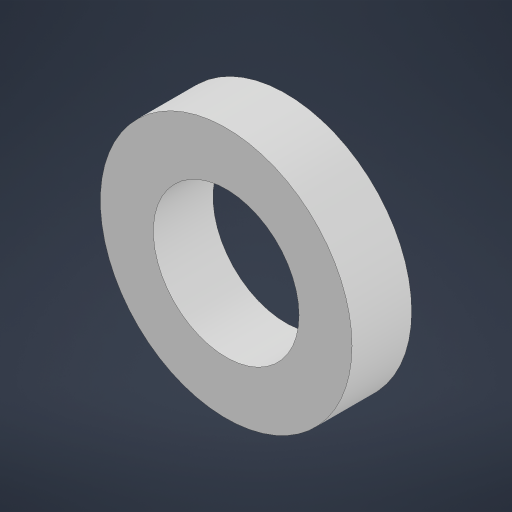
# Autodesk Inventor part: counterbore side
Saved by Autodesk Inventor 2023.2 (Build 272271030, 271C)
## iProperties
Created: 2023-04-05
Part Number: counterbore side
Material: Generic
Document SubType Name: Modeling
Designer: ralph
Density: 1 g/cm^3
Appearance: Default
Author: ralph
Autodesk Inventor part; units mm, degrees
ref_plane "YZ Plane" through (0, 0, 0) normal (1, 0, 0) x (0, 1, 0)
ref_plane "XZ Plane" through (0, 0, 0) normal (0, 1, 0) x (-1, 0, 0)
ref_plane "XY Plane" through (0, 0, 0) normal (0, 0, 1) x (1, 0, 0)
sketch "Sketch1" plane through (0, 0, 0) normal (0, 0, 1) x (1, 0, 0)
  arc A0 (13.9214, 24.4216) -> (10.9603, 25.6482) centre (0, -5) ccw projected
  arc A1 (9.0874, 23.6613) -> (10.9603, 25.6482) centre (2.0185, 32.201) ccw projected
  arc A2 (2.5726, 24.9572) -> (9.0874, 23.6613) centre (6.35, 26.9236) ccw projected
  arc A3 (1.6025, 27.5096) -> (2.5726, 24.9572) centre (12.3713, 30.1417) ccw projected
  arc A4 (1.6025, 27.5096) -> (-1.6025, 27.5096) centre (0, -5) ccw projected
  arc A5 (-2.5726, 24.9572) -> (-1.6025, 27.5096) centre (-12.3713, 30.1417) ccw projected
  arc A6 (-9.0874, 23.6613) -> (-2.5726, 24.9572) centre (-6.35, 26.9236) ccw projected
  arc A7 (-10.9603, 25.6482) -> (-9.0874, 23.6613) centre (-2.0185, 32.201) ccw projected
  arc A8 (-10.9603, 25.6482) -> (-13.9214, 24.4216) centre (0, -5) ccw projected
  arc A9 (-13.8408, 21.6924) -> (-13.9214, 24.4216) centre (-24.8777, 22.7324) ccw projected
  arc A10 (-19.3639, 18.002) -> (-13.8408, 21.6924) centre (-18.0833, 22.0635) ccw projected
  arc A11 (-21.8546, 19.1209) -> (-19.3639, 18.002) centre (-16.1011, 28.5967) ccw projected
  arc A12 (-21.8546, 19.1209) -> (-24.1209, 16.8546) centre (0, -5) ccw projected
  arc A13 (-23.002, 14.3639) -> (-24.1209, 16.8546) centre (-33.5967, 11.1011) ccw projected
  arc A14 (-26.6924, 8.8408) -> (-23.002, 14.3639) centre (-27.0635, 13.0833) ccw projected
  arc A15 (-29.4216, 8.9214) -> (-26.6924, 8.8408) centre (-27.7324, 19.8777) ccw projected
  arc A16 (-29.4216, 8.9214) -> (-30.6482, 5.9603) centre (0, -5) ccw projected
  arc A17 (-28.6613, 4.0874) -> (-30.6482, 5.9603) centre (-37.201, -2.9815) ccw projected
  arc A18 (-29.9572, -2.4274) -> (-28.6613, 4.0874) centre (-31.9236, 1.35) ccw projected
  arc A19 (-32.5096, -3.3975) -> (-29.9572, -2.4274) centre (-35.1417, 7.3713) ccw projected
  arc A20 (-32.5096, -3.3975) -> (-32.5096, -6.6025) centre (0, -5) ccw projected
  arc A21 (-29.9572, -7.5726) -> (-32.5096, -6.6025) centre (-35.1417, -17.3713) ccw projected
  arc A22 (-28.6613, -14.0874) -> (-29.9572, -7.5726) centre (-31.9236, -11.35) ccw projected
  arc A23 (-30.6482, -15.9603) -> (-28.6613, -14.0874) centre (-37.201, -7.0185) ccw projected
  arc A24 (-30.6482, -15.9603) -> (-29.4216, -18.9214) centre (0, -5) ccw projected
  arc A25 (-26.6924, -18.8408) -> (-29.4216, -18.9214) centre (-27.7324, -29.8777) ccw projected
  arc A26 (-23.002, -24.3639) -> (-26.6924, -18.8408) centre (-27.0635, -23.0833) ccw projected
  arc A27 (-24.1209, -26.8546) -> (-23.002, -24.3639) centre (-33.5967, -21.1011) ccw projected
  arc A28 (-24.1209, -26.8546) -> (-21.8546, -29.1209) centre (0, -5) ccw projected
  arc A29 (-19.3639, -28.002) -> (-21.8546, -29.1209) centre (-16.1011, -38.5967) ccw projected
  arc A30 (-13.8408, -31.6924) -> (-19.3639, -28.002) centre (-18.0833, -32.0635) ccw projected
  arc A31 (-13.9214, -34.4216) -> (-13.8408, -31.6924) centre (-24.8777, -32.7324) ccw projected
  arc A32 (-13.9214, -34.4216) -> (-10.9603, -35.6482) centre (0, -5) ccw projected
  arc A33 (-9.0874, -33.6613) -> (-10.9603, -35.6482) centre (-2.0185, -42.201) ccw projected
  arc A34 (-2.5726, -34.9572) -> (-9.0874, -33.6613) centre (-6.35, -36.9236) ccw projected
  arc A35 (-1.6025, -37.5096) -> (-2.5726, -34.9572) centre (-12.3713, -40.1417) ccw projected
  arc A36 (-1.6025, -37.5096) -> (1.6025, -37.5096) centre (0, -5) ccw projected
  arc A37 (2.5726, -34.9572) -> (1.6025, -37.5096) centre (12.3713, -40.1417) ccw projected
  arc A38 (9.0874, -33.6613) -> (2.5726, -34.9572) centre (6.35, -36.9236) ccw projected
  arc A39 (10.9603, -35.6482) -> (9.0874, -33.6613) centre (2.0185, -42.201) ccw projected
  arc A40 (10.9603, -35.6482) -> (13.9214, -34.4216) centre (0, -5) ccw projected
  arc A41 (13.8408, -31.6924) -> (13.9214, -34.4216) centre (24.8777, -32.7324) ccw projected
  arc A42 (19.3639, -28.002) -> (13.8408, -31.6924) centre (18.0833, -32.0635) ccw projected
  arc A43 (21.8546, -29.1209) -> (19.3639, -28.002) centre (16.1011, -38.5967) ccw projected
  arc A44 (21.8546, -29.1209) -> (24.1209, -26.8546) centre (0, -5) ccw projected
  arc A45 (23.002, -24.3639) -> (24.1209, -26.8546) centre (33.5967, -21.1011) ccw projected
  arc A46 (26.6924, -18.8408) -> (23.002, -24.3639) centre (27.0635, -23.0833) ccw projected
  arc A47 (29.4216, -18.9214) -> (26.6924, -18.8408) centre (27.7324, -29.8777) ccw projected
  arc A48 (29.4216, -18.9214) -> (30.6482, -15.9603) centre (0, -5) ccw projected
  arc A49 (28.6613, -14.0874) -> (30.6482, -15.9603) centre (37.201, -7.0185) ccw projected
  arc A50 (29.9572, -7.5726) -> (28.6613, -14.0874) centre (31.9236, -11.35) ccw projected
  arc A51 (32.5096, -6.6025) -> (29.9572, -7.5726) centre (35.1417, -17.3713) ccw projected
  arc A52 (32.5096, -6.6025) -> (32.5096, -3.3975) centre (0, -5) ccw projected
  arc A53 (29.9572, -2.4274) -> (32.5096, -3.3975) centre (35.1417, 7.3713) ccw projected
  arc A54 (28.6613, 4.0874) -> (29.9572, -2.4274) centre (31.9236, 1.35) ccw projected
  arc A55 (30.6482, 5.9603) -> (28.6613, 4.0874) centre (37.201, -2.9815) ccw projected
  arc A56 (30.6482, 5.9603) -> (29.4216, 8.9214) centre (0, -5) ccw projected
  arc A57 (26.6924, 8.8408) -> (29.4216, 8.9214) centre (27.7324, 19.8777) ccw projected
  arc A58 (23.002, 14.3639) -> (26.6924, 8.8408) centre (27.0635, 13.0833) ccw projected
  arc A59 (24.1209, 16.8546) -> (23.002, 14.3639) centre (33.5967, 11.1011) ccw projected
  arc A60 (24.1209, 16.8546) -> (21.8546, 19.1209) centre (0, -5) ccw projected
  arc A61 (19.3639, 18.002) -> (21.8546, 19.1209) centre (16.1011, 28.5967) ccw projected
  arc A62 (13.8408, 21.6924) -> (19.3639, 18.002) centre (18.0833, 22.0635) ccw projected
  arc A63 (13.9214, 24.4216) -> (13.8408, 21.6924) centre (24.8777, 22.7324) ccw projected
  circle A64 centre (0, -5) radius 24.13
  circle A65 centre (0, -5) radius 13.97 projected
  circle A66 centre (0, 14.05) radius 2.3813 projected
  circle A67 centre (19.05, -5) radius 2.3813 projected
  circle A68 centre (-19.05, -5) radius 2.3813 projected
  circle A69 centre (0, -24.05) radius 2.3813 projected
  point P0 (0, 0)
  dimension "d0" = 48.26
  constraints: 1 centre point, 1 coincident
  measures "d0" diameter of A64
extrude "Extrusion1" add sketch "Sketch1" along normal blind 9.525 contours A64 | A65 | A66 | A67 | A68 | A69
sketch "Sketch2" plane through (0, -5, 9.525) normal (0, 0, 1) x (1, 0, 0)
  circle A0 centre (0, 0) radius 24.13 projected
  circle A1 centre (0, 19.05) radius 4.7625
  circle A2 centre (-19.05, 0) radius 1.27 projected
  circle A3 centre (-19.05, 0) radius 4.7625
  circle A4 centre (19.05, 0) radius 4.7625
  circle A5 centre (0, -19.05) radius 4.7625
  point P0 (0, 5)
  dimension "d3" = 9.525
  dimension "d4" = 9.525
  dimension "d5" = 9.525
  dimension "d6" = 9.525
  constraints: 4 centre point, 1 coincident
  measures "d3" diameter of A1
  measures "d4" diameter of A3
  measures "d5" diameter of A4
  measures "d6" diameter of A5
ref_plane "Work Plane1" through (-23.0187, -8.9687, 4.5858) normal (0, 0, -1) x (0, 1, 0)
extrude "Extrusion2" [suppressed]
sketch "Sketch3" plane through (0, -5, 9.525) normal (0, 0, 1) x (1, 0, 0)
  circle A0 centre (0, 0) radius 13.97
  point P0 (0, 5)
  dimension "d9" = 27.94
  constraints: 1 centre point
  measures "d9" diameter of A0
extrude "Extrusion3" cut sketch "Sketch3" against normal blind 39.6875
sketch "Sketch4" plane through (0, -5, 9.525) normal (0, 0, 1) x (1, 0, 0)
  circle A0 centre (0, 0) radius 13.97 projected
  circle A1 centre (0, 0) radius 24.13 projected
  point P0 (0, 5)
extrude "Extrusion4" add sketch "Sketch4" against normal blind 11.43
body "Solid1"
